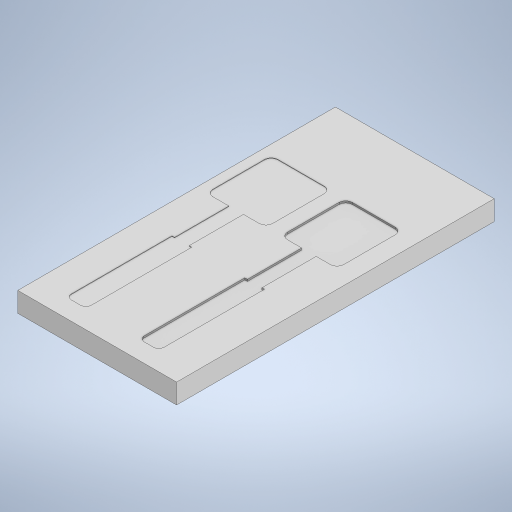
# Autodesk Inventor part: 0p03_total_thickness
Saved by Autodesk Inventor 2024.2 (Build 282272000, 272)
## iProperties
Created: 2024-10-29
Part Number: 0p03_total_thickness
Material: Generic
Document SubType Name: Modeling
Designer: Tom
Density: 1 g/cm^3
Appearance: Default
Author: Tom
Autodesk Inventor part; units mm, degrees
ref_plane "YZ Plane" through (0, 0, 0) normal (1, 0, 0) x (0, 1, 0)
ref_plane "XZ Plane" through (0, 0, 0) normal (0, 1, 0) x (-1, 0, 0)
ref_plane "XY Plane" through (0, 0, 0) normal (0, 0, 1) x (1, 0, 0)
sketch "Sketch1" plane through (0, 0, 0) normal (0, 1, 0) x (-1, 0, 0)
  line L0 (0, 0) -> (76.2, 0)
  line L1 (76.2, 0) -> (76.2, -152.4)
  line L2 (76.2, -152.4) -> (0, -152.4)
  line L3 (0, -152.4) -> (0, 0)
  dimension "d0" = 76.2
  dimension "d1" = 152.4
  constraints: 8 end point, 2 parallel, 1 horizontal, 1 perpendicular
  measures "d0" distance of L0.start L0.end
  measures "d1" distance of L2.end L0.start
extrude "Extrusion1" add sketch "Sketch1" along normal blind 9.525
sketch "Sketch2" plane through (0, 9.525, 0) normal (0, 1, 0) x (1, 0, 0)
  line L0 (-59.5312, 8.89) -> (-54.7688, 8.89)
  line L1 (-52.3875, 11.2712) -> (-52.3875, 59.5312)
  line L2 (-61.9125, 59.5312) -> (-61.9125, 11.2712)
  line L3 (-76.2, 152.4) -> (-76.2, 0) projected
  line L4 (-76.2, 0) -> (0, 0) projected
  arc A0 (-61.9125, 9.0487) -> (-61.7538, 8.89) centre (-61.7538, 9.0487) ccw
  arc A1 (-52.5462, 8.89) -> (-52.3875, 9.0487) centre (-52.5462, 9.0487) ccw
  arc A2 (-52.3875, 59.5312) -> (-52.5462, 59.69) centre (-52.5462, 59.5312) ccw
  arc A3 (-61.7538, 59.69) -> (-61.9125, 59.5312) centre (-61.7538, 59.5312) ccw
  line L5 (-60.6425, 59.69) -> (-53.6575, 59.69)
  line L6 (-53.6575, 59.69) -> (-53.6575, 116.84)
  line L7 (-60.6425, 116.84) -> (-60.6425, 59.69)
  line L8 (-52.5462, 59.69) -> (-53.6575, 59.69)
  line L9 (-60.6425, 59.69) -> (-61.7538, 59.69)
  line L10 (-68.2625, 116.84) -> (-46.0375, 116.84)
  line L11 (-42.8625, 113.665) -> (-42.8625, 88.9)
  line L12 (-46.0375, 85.725) -> (-68.2625, 85.725)
  line L13 (-71.4375, 88.9) -> (-71.4375, 113.665)
  arc A4 (-71.4375, 88.9) -> (-68.2625, 85.725) centre (-68.2625, 88.9) ccw
  arc A5 (-68.2625, 116.84) -> (-71.4375, 113.665) centre (-68.2625, 113.665) ccw
  arc A6 (-42.8625, 113.665) -> (-46.0375, 116.84) centre (-46.0375, 113.665) ccw
  arc A7 (-46.0375, 85.725) -> (-42.8625, 88.9) centre (-46.0375, 88.9) ccw
  arc A8 (-54.7688, 8.89) -> (-52.3875, 11.2712) centre (-54.7688, 11.2712) ccw
  arc A9 (-61.9125, 11.2712) -> (-59.5312, 8.89) centre (-59.5312, 11.2712) ccw
  point P0 (-61.9125, 8.89)
  point P1 (-52.3875, 69.85)
  point P2 (-52.3875, 8.89)
  point P3 (-61.9125, 69.85)
  point P4 (-57.15, 69.85)
  point P5 (-57.15, 132.715)
  point P6 (-71.4375, 116.84)
  point P7 (-42.8625, 85.725)
  point P8 (-42.8625, 116.84)
  point P9 (-71.4375, 85.725)
  point P10 (-57.15, 116.84)
  point P11 (-57.15, 8.89)
  point P12 (-57.15, 59.69)
  point P13 (-60.6425, 85.725)
  point P14 (-53.6575, 85.725)
  dimension "d22" = 0
  dimension "d28" = 0
  dimension "d36" = 26.035
  dimension "d37" = 50.8
  dimension "d41" = 9.525
  dimension "d47" = 2.3813
  constraints: 24 end point, 22 tangent, 20 point on circle, 20 point on line, 10 centre point, 7 equal radius, 6 parallel, 3 horizontal, 3 midpoint, 3 perpendicular
  measures "d22" horizontal distance of point (-57.15, 69.85) point (-57.15, 132.715)
  measures "d28" horizontal distance of point (-57.15, 8.89) point (-57.15, 59.69)
  measures "d36" distance between parallel lines of L5 L12
  measures "d37" distance between parallel lines of L0 L5
  measures "d41" distance between parallel lines of L2 L1
  measures "d47" radius of A8
extrude "Extrusion2" cut sketch "Sketch2" against normal blind 0.254
sketch "Sketch3" plane through (0, 9.525, 0) normal (0, 1, 0) x (1, 0, 0)
  line L0 (-24.6057, 8.9288) -> (-19.8432, 8.9288)
  line L1 (-17.4619, 11.31) -> (-17.4619, 57.3087)
  line L2 (-26.9869, 57.3087) -> (-26.9869, 11.31)
  arc A0 (-26.9869, 11.31) -> (-24.6057, 8.9288) centre (-24.6057, 11.31) ccw
  arc A1 (-19.8432, 8.9288) -> (-17.4619, 11.31) centre (-19.8432, 11.31) ccw
  line L3 (-18.7319, 59.69) -> (-18.7319, 116.84)
  line L4 (-25.7169, 116.84) -> (-25.7169, 59.69)
  line L5 (0, 152.4) -> (-76.2, 152.4) projected
  line L6 (-32.5432, 116.84) -> (-11.9057, 116.84)
  line L7 (-8.7307, 113.665) -> (-8.7307, 88.9)
  line L8 (-11.9057, 85.725) -> (-32.5432, 85.725)
  line L9 (-35.7182, 88.9) -> (-35.7182, 113.665)
  line L10 (-46.0375, 85.725) -> (-53.6575, 85.725) projected
  arc A2 (-32.5432, 116.84) -> (-35.7182, 113.665) centre (-32.5432, 113.665) ccw
  arc A3 (-35.7182, 88.9) -> (-32.5432, 85.725) centre (-32.5432, 88.9) ccw
  arc A4 (-11.9057, 85.725) -> (-8.7307, 88.9) centre (-11.9057, 88.9) ccw
  arc A5 (-8.7307, 113.665) -> (-11.9057, 116.84) centre (-11.9057, 113.665) ccw
  line L11 (-17.4619, 57.3087) -> (-17.4619, 59.69)
  line L12 (-17.4619, 59.69) -> (-18.7319, 59.69)
  line L13 (-25.7169, 59.69) -> (-26.9869, 59.69)
  line L14 (-26.9869, 59.69) -> (-26.9869, 57.3087)
  point P0 (0, 0)
  point P1 (-26.9869, 8.9288)
  point P2 (-21.4307, 55.0791)
  point P3 (-22.2244, 132.715)
  point P4 (-8.7307, 85.725)
  point P5 (-35.7182, 85.725)
  point P6 (-22.2244, 116.84)
  point P7 (-49.8475, 85.725)
  point P8 (-25.7169, 85.725)
  point P9 (-18.7319, 116.84)
  point P10 (-18.7319, 85.725)
  point P11 (-25.1613, 59.69)
  point P12 (-22.2244, 8.9288)
  dimension "d12" = 9.525
  dimension "d13" = 2.3813
  dimension "d33" = 0
  dimension "d34" = 3.175
  dimension "d40" = 26.035
  dimension "d42" = 0
  dimension "d43" = 0
  dimension "d45" = 6.985
  constraints: 26 end point, 12 point on circle, 12 tangent, 8 point on line, 6 centre point, 4 equal radius, 4 parallel, 4 perpendicular, 3 horizontal, 3 midpoint, 1 vertical
  measures "d12" distance between parallel lines of L1 L2
  measures "d13" radius of A0
  measures "d33" distance from line of point (-49.847, 85.725) L8
  measures "d34" radius of A2
  measures "d40" distance from line of L8 point (-25.161, 59.69)
  measures "d42" horizontal distance of point (-22.224, 132.715) point (-22.224, 8.929)
  measures "d43" horizontal distance of point (-22.224, 116.84) point (-22.224, 132.715)
  measures "d45" distance between parallel lines of L3 L4
extrude "Extrusion3" cut sketch "Sketch3" against normal blind 0.889
body "Solid1"
